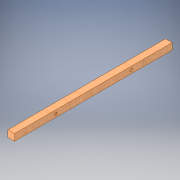
# Autodesk Inventor part: Spacer
Saved by Autodesk Inventor 2019.3 (Build 233278000, 278)
## iProperties
Created: 2019-01-17
Part Number: Spacer
Material: Holz (Eiche)
Document SubType Name: Modeling
Designer: Jonas
Density: 0.76 g/cm^3
Appearance: Kirsche - natur - schwacher Glanz
Author: Jonas
Autodesk Inventor part; units mm, degrees
ref_plane "YZ Plane" through (0, 0, 0) normal (1, 0, 0) x (0, 1, 0)
ref_plane "XZ Plane" through (0, 0, 0) normal (0, 1, 0) x (-1, 0, 0)
ref_plane "XY Plane" through (0, 0, 0) normal (0, 0, 1) x (1, 0, 0)
sketch "Skizze1" plane through (0, 0, 0) normal (0, 1, 0) x (-1, 0, 0)
  line L0 (-5, 120) -> (5, 120)
  line L1 (5, 120) -> (5, -120)
  line L2 (5, -120) -> (-5, -120)
  line L3 (-5, -120) -> (-5, 120)
  line L4 (-5, 120) -> (5, -120) construction
  line L5 (5, 120) -> (-5, -120) construction
  point P0 (0, 0)
  dimension "d0" = 240
  dimension "d1" = 10
  constraints: 12 end point, 2 midpoint, 2 parallel, 1 horizontal, 1 perpendicular
  measures "d0" distance of L0.end L1.end
  measures "d1" distance of L1.end L2.end
extrude "Extrusion1" add sketch "Skizze1" along normal blind 10
sketch "Skizze2" plane through (5, 0, 120) normal (1, 0, 0) x (0, 0, -1)
  line L0 (0, 0) -> (0, 10) projected
  line L1 (0, 5) -> (250, 5)
  line L2 (240, 0) -> (240, 10) projected
  point P0 (120, 0)
  point P1 (62.5, 5)
  point P2 (177.5, 5)
  dimension "d4" = 62.5
  dimension "d5" = 62.5
  constraints: 2 end point, 2 point on line, 1 horizontal, 1 midpoint, 1 other
  measures "d4" distance from line of L0 point (62.5, 5)
hole "Bohrung1" at (5, 5, -57.5) at (5, 5, 57.5) direction (-1, 0, 0) diameter 3 end through all countersink diameter 4 countersink angle 90
